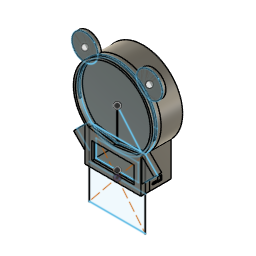
Data-visualization v7 (Autodesk Fusion 360 design; units mm, degrees)
Autodesk Fusion 360 part; units mm, degrees
sketch "Sketch1" plane through (0, 0, 0) normal (0, 1, 0) x (1, 0, 0)
  line L0 (49, -55) -> (-49, -55)
  line L1 (0, -15) -> (49, -15)
  line L2 (0, -15) -> (-49, -15)
  line L3 (-49, -55) -> (-49, -15)
  line L4 (49, -15) -> (49, -55)
  line L5 (65, -80) -> (-65, -80)
  line L6 (-65, -80) -> (-65, 80)
  line L7 (-65, 80) -> (65, 80)
  line L8 (65, 80) -> (65, -80)
  line L9 (65, -80) -> (-65, 80) construction
  line L10 (-65, -80) -> (65, 80) construction
  line L11 (0, -80) -> (0, -145)
  line L12 (0, -70) -> (65, -80)
  line L13 (0, -70) -> (-65, -80)
  circle A0 centre (0, -145) radius 91.9239
  line L14 (-65, 0) -> (65, 0)
  circle A1 centre (0, -145) radius 86.9239
  line L15 (65, -80) -> (93.2843, -51.7157)
  line L16 (93.2843, -51.7157) -> (65, -23.4315)
  line L17 (-65, -80) -> (-93.2843, -51.7157)
  line L18 (-93.2843, -51.7157) -> (-65, -23.4315)
  circle A2 centre (-75, -225) radius 30
  circle A3 centre (75, -225) radius 30
  circle A4 centre (0, -145) radius 2.5
  line L19 (0, -145) -> (0, -70)
  line L20 (0, -145) -> (56.14, -78.6369)
  point P0 (0, -15)
  dimension "d2" = 130
  dimension "d3" = 65
  dimension "d6" = -5
  dimension "d9" = 40
  dimension "d13" = 60
  dimension "d14" = 60
  dimension "d29" = 5
  constraint horizontal L0
  constraint coincident P0 L1.start
  constraint perpendicular L2 L3
  constraint perpendicular L0 L4
  constraint horizontal L5
  constraint perpendicular L5 L6
  constraint parallel L5 L7
  constraint parallel L6 L8
  constraint coincident L9 origin
  constraint coincident L10 origin
  constraint midpoint L5 L11.start
  constraint perpendicular L5 L11
  constraint coincident L11.end A0.centre
  constraint coincident L5.start A0
  constraint midpoint L6 L14.start
  constraint midpoint L8 L14.end
  constraint coincident L8 L16.end
  constraint perpendicular L15 L16
  constraint parallel L16 L17
  constraint coincident L6 L18.end
  constraint perpendicular L17 L18
  constraint concentric A0 A4
  constraint parallel L11 L19
  constraint coincident L12 L20.end
  constraint coincident A1 L20.end
  measures "d2" distance of L6.end L7.end
  measures "d3" distance of L11.start L11.end
  measures "d9" distance of L5.start L15.end
  measures "d13" diameter of A2
  measures "d14" diameter of A3
  measures "d29" diameter of A4
extrude "Extrude1" add sketch "Sketch1" along normal blind 10 contours L0 L1 L2 L3 L4 L6 L8 A0 L14 | L0 L12 L13 A0 A1 | L5 A0 A1 A3 | L5 L12 A1 | L5 L13 A1 | L5 A0 A1 A2 | L5 L11 A1 A2 A3 A4 L19 L20 | L5 A1 L20 | L5 L12 L19 L20 | L12 L13 A1 | L5 L13 A1 L19 | A0 A1 A2 | L5 L11 A4 L19 L20 | A0 A1 A3 | A1 A2 | A0 A1 A2 A3 | L11 A4 L19 L20 | L11 A4 L19 L20 | A1 A3 makes body 1
extrude "Extrude2" cut sketch "Sketch1" along normal blind 6 contours L5 L11 A1 A2 A3 A4 L19 L20 | L5 L11 A4 L19 L20 | A1 A2 | L11 A4 L19 L20 | L11 A4 L19 L20 | A1 A3 bodies 1
extrude "Extrude3" add sketch "Sketch1" along normal blind 10 contours L8 L15 L16 | L6 L17 L18 bodies 1
extrude "Extrude4" add sketch "Sketch1" along normal blind 6 contours A0 A3 bodies 1
extrude "Extrude5" add sketch "Sketch1" along normal blind 6 contours A0 A2 bodies 1
extrude "Extrude6" cut sketch "Sketch1" along normal blind 6 contours L5 A1 L20 | L5 L12 L19 L20 | L5 L13 A1 L19 bodies 1
extrude "Extrude7" add sketch "Sketch1" against normal blind 10 contours L0 L1 L2 L3 L4 L6 L8 A0 L14 | L0 L12 L13 A0 A1 | L5 A0 A1 A3 | L5 L12 A1 | L5 L13 A1 | L5 A0 A1 A2 | A0 A1 A2 | A0 A1 A3 | A0 A1 A2 A3 bodies 1
extrude "Extrude8" add sketch "Sketch1" against normal blind 10 contours L12 L13 A1 bodies 1
sketch "Sketch2" plane through (0, 0, 360) normal (0, 0, -1) x (1, 0, 0)
  line L0 (-200, 0) -> (200, 0)
  line L1 (200, 0) -> (200, 4.5)
  line L2 (200, 4.5) -> (-200, 4.5)
  line L3 (-200, 4.5) -> (-200, 0)
  line L4 (-200, 4.5) -> (200, 4.5)
  line L5 (200, 4.5) -> (200, 0)
  line L6 (200, 0) -> (-200, 0)
  line L7 (-200, 0) -> (-200, 4.5)
  constraint horizontal L4
  constraint vertical L5
  constraint horizontal L6
  constraint vertical L7
  constraint coincident L0.end L1.start
  constraint coincident L2.end L3.start
extrude "Extrude10" cut sketch "Sketch2" along normal blind 240 bodies 1
extrude "Extrude11" cut sketch "Sketch1" along normal blind 10 contours L11 A4 L19 L20 | L11 A4 L19 L20 bodies 1
extrude "Extrude12" add sketch "Sketch1" against normal blind 8 contours L8 L15 L16 bodies 1
extrude "Extrude13" add sketch "Sketch1" against normal blind 8 contours L6 L17 L18 bodies 1
sketch "Sketch4" plane through (0, 10, 0) normal (0, 1, 0) x (-1, 0, 0)
  circle A0 centre (0, 145) radius 2.5
  line L0 (49, 15) -> (-49, 15)
  line L1 (-49, 15) -> (-49, 55)
  line L2 (-49, 55) -> (49, 55)
  line L3 (49, 55) -> (49, 15)
  arc A1 (65, 80) -> (-65, 80) centre (0, 145) ccw
  line L4 (-65, 80) -> (-93.2843, 51.7157)
  line L5 (-93.2843, 51.7157) -> (-65, 23.4315)
  line L6 (-65, 23.4315) -> (-65, 0)
  line L7 (-65, 0) -> (65, 0)
  line L8 (65, 0) -> (65, 23.4315)
  line L9 (65, 23.4315) -> (93.2843, 51.7157)
  line L10 (93.2843, 51.7157) -> (65, 80)
  line L11 (-65, 80) -> (65, 80)
  line L12 (65, 80) -> (65, 0)
  line L13 (65, 0) -> (-65, 0)
  line L14 (-65, 0) -> (-65, 80)
  circle A2 centre (0, 145) radius 91.9239
  constraint horizontal L11
  constraint vertical L12
  constraint horizontal L13
  constraint vertical L14
  constraint coincident L7.end L8.start
  constraint coincident A1.end L4.start
  constraint concentric A0 A2
extrude "Extrude14" add sketch "Sketch4" along normal blind 50 separate body contours L0 L1 L2 L3 L6 L7 L8 L12 L13 L14 A2 | L0 L1 L2 L3 A2 | L2 A2 | L2 L11 A2 | A1 L11 A2 makes body 2
move_face "OffsetFaces1" offset 50 1 faces at (-2.4504, 43.3333, 144.5046) on bodies 2
sketch "Sketch5" plane through (0, 10, 0) normal (0, -1, 0) x (1, 0, 0)
  line L0 (-65, 80) -> (-65, 0)
  line L1 (-65, 0) -> (65, 0)
  line L2 (65, 0) -> (65, 80)
  arc A0 (65, 80) -> (-65, 80) centre (0, 145) ccw
  circle A1 centre (0, 145) radius 85
  line L3 (-60, 84.792) -> (-60, 5)
  line L4 (-60, 84.792) -> (60, 84.792)
  line L5 (60, 84.792) -> (60, 5)
  line L6 (60, 5) -> (-60, 5)
  line L7 (-60, 5) -> (-60, 84.792)
  dimension "d39" = 170
  dimension "d40" = -5
  constraint concentric A0 A1
  constraint coincident A1 L3.start
  constraint horizontal L4
  constraint vertical L5
  constraint horizontal L6
  constraint vertical L7
  measures "d39" diameter of A1
extrude "Extrude15" cut sketch "Sketch5" against normal blind 45 contours A1 L4 picked at (-9.4952, 166.9681) bodies 2
extrude "Extrude16" cut sketch "Sketch5" against normal blind 45 contours A1 L4 | A1 L3 L5 L6 L7 picked at (16.9474, 82.1553) bodies 2
sketch "Sketch6" plane through (0, 10, 0) normal (0, 1, 0) x (-1, 0, 0)
  circle A0 centre (0, 145) radius 2.5
  line L0 (49, 15) -> (-49, 15)
  line L1 (-49, 15) -> (-49, 55)
  line L2 (-49, 55) -> (49, 55)
  line L3 (49, 55) -> (49, 15)
  arc A1 (65, 80) -> (-65, 80) centre (0, 145) ccw
  line L4 (-65, 80) -> (-93.2843, 51.7157)
  line L5 (-93.2843, 51.7157) -> (-65, 23.4315)
  line L6 (-65, 23.4315) -> (-65, 0)
  line L7 (-65, 0) -> (65, 0)
  line L8 (65, 0) -> (65, 23.4315)
  line L9 (65, 23.4315) -> (93.2843, 51.7157)
  line L10 (93.2843, 51.7157) -> (65, 80)
  line L11 (65, 0) -> (-65, 0)
  line L12 (-65, 0) -> (-65, 80)
  line L13 (-65, 80) -> (65, 80)
  line L14 (65, 80) -> (65, 0)
  line L15 (61, 4) -> (-61, 4)
  line L16 (-61, 4) -> (-61, 76)
  line L17 (-61, 76) -> (61, 76)
  line L18 (61, 76) -> (61, 4)
  line L19 (0, 66) -> (61, 66)
  line L20 (0, 66) -> (-61, 66)
  line L21 (-65, 70) -> (65, 70)
  line L22 (-65, 70) -> (-62, 70)
  line L23 (-62, 70) -> (-62, 34)
  line L24 (-62, 34) -> (-65, 34)
  line L25 (-65, 34) -> (-65, 70)
  line L26 (65, 70) -> (62, 70)
  line L27 (62, 70) -> (62, 34)
  line L28 (62, 34) -> (65, 34)
  line L29 (65, 34) -> (65, 70)
  dimension "d45" = 4
  dimension "d52" = 3
  dimension "d53" = 36
  dimension "d54" = 3
  dimension "d55" = 36
  constraint horizontal L11
  constraint vertical L12
  constraint horizontal L13
  constraint vertical L14
  constraint coincident A1.end L4.start
  constraint coincident L7.end L8.start
  constraint coincident L18 L19.end
  constraint perpendicular L18 L19
  constraint coincident L16 L20.end
  constraint perpendicular L16 L20
  constraint coincident L12 L21.start
  constraint coincident L14 L21.end
  constraint perpendicular L14 L21
  constraint horizontal L22
  constraint vertical L23
  constraint horizontal L24
  constraint vertical L25
  constraint horizontal L26
  constraint vertical L27
  constraint horizontal L28
  constraint vertical L29
  measures "d52" distance of L21.start L22.end
  measures "d53" distance of L21.start L24.end
  measures "d8" distance of L21.end L26.end
  measures "d8" distance of L21.end L28.end
extrude "Extrude17" cut sketch "Sketch6" against normal blind 15 contours L15 L16 L18 L19 L20 bodies 1
extrude "Extrude18" cut sketch "Sketch6" against normal blind 10 contours L14 L21 L26 L27 L28 L29 | L12 L21 L22 L23 L24 L25 bodies 1
extrude "Extrude19" add sketch "Sketch6" against normal blind 9.9 contours L14 L21 L26 L27 L28 L29 | L12 L21 L22 L23 L24 L25 bodies 2
move_face "OffsetFaces2" offset -0.2 1 faces at (-65, 6.6667, 58) on bodies 1
sketch "Sketch7" plane through (65, 0, 0) normal (1, 0, 0) x (0, 1, 0)
  line L0 (10, 34) -> (10, 0)
  line L1 (10, 0) -> (60, 0)
  line L2 (60, 0) -> (60, 80)
  line L3 (60, 80) -> (10, 80)
  line L4 (10, 80) -> (10, 70)
  line L5 (10, 70) -> (0.1, 70)
  line L6 (0.1, 70) -> (0.1, 34)
  line L7 (0.1, 34) -> (10, 34)
  line L8 (38.3, 19.65) -> (29.1, 19.65)
  line L9 (29.1, 19.65) -> (29.1, 8.45)
  line L10 (29.1, 8.45) -> (38.3, 8.45)
  line L11 (38.3, 8.45) -> (38.3, 19.65)
  line L12 (38.3, 19.65) -> (29.1, 8.45) construction
  line L13 (29.1, 19.65) -> (38.3, 8.45) construction
  line L14 (27.8, 14.05) -> (16.2, 14.05)
  line L15 (16.2, 14.05) -> (16.2, 9.25)
  line L16 (16.2, 9.25) -> (27.8, 9.25)
  line L17 (27.8, 9.25) -> (27.8, 14.05)
  line L18 (27.8, 14.05) -> (16.2, 9.25) construction
  line L19 (16.2, 14.05) -> (27.8, 9.25) construction
  point P0 (33.7, 14.05)
  point P1 (22, 11.65)
  dimension "d71" = 9.2
  dimension "d72" = 11.2
  dimension "d73" = 11.6
  dimension "d74" = 4.8
  constraint horizontal L8
  constraint perpendicular L8 L9
  constraint parallel L8 L10
  constraint parallel L9 L11
  constraint coincident L12 P0
  constraint coincident L13 P0
  constraint horizontal L14
  constraint perpendicular L14 L15
  constraint parallel L14 L16
  constraint parallel L15 L17
  constraint coincident L18 P1
  constraint coincident L19 P1
  measures "d71" distance of L9.end L10.end
  measures "d72" distance of L8.end L9.end
  measures "d73" distance of L15.end L16.end
  measures "d74" distance of L14.end L15.end
extrude "Extrude20" cut sketch "Sketch7" against normal blind 5 contours L8 L9 L10 L11 | L14 L15 L16 L17 bodies 2
fillet "Fillet1" radius 0.5 4 edges at (62.5, 38.3, 19.65) (62.5, 38.3, 8.45) (62.5, 29.1, 8.45) (62.5, 29.1, 19.65) on bodies 2
fillet "Fillet2" radius 1.8 4 edges at (62.5, 27.8, 14.05) (62.5, 27.8, 9.25) (62.5, 16.2, 14.05) (62.5, 16.2, 9.25) on bodies 2
sketch "Sketch8" plane through (60, 0, 0) normal (-1, 0, 0) x (0, -1, 0)
  line L0 (-37.8, 19.65) -> (-29.6, 19.65)
  arc A0 (-29.1, 19.15) -> (-29.6, 19.65) centre (-29.6, 19.15) ccw
  line L1 (-29.1, 19.15) -> (-29.1, 8.95)
  arc A1 (-29.6, 8.45) -> (-29.1, 8.95) centre (-29.6, 8.95) ccw
  line L2 (-29.6, 8.45) -> (-37.8, 8.45)
  arc A2 (-38.3, 8.95) -> (-37.8, 8.45) centre (-37.8, 8.95) ccw
  line L3 (-38.3, 8.95) -> (-38.3, 19.15)
  arc A3 (-37.8, 19.65) -> (-38.3, 19.15) centre (-37.8, 19.15) ccw
  line L4 (-26, 14.05) -> (-18, 14.05)
  arc A4 (-16.2, 12.25) -> (-18, 14.05) centre (-18, 12.25) ccw
  line L5 (-16.2, 12.25) -> (-16.2, 11.05)
  arc A5 (-18, 9.25) -> (-16.2, 11.05) centre (-18, 11.05) ccw
  line L6 (-18, 9.25) -> (-26, 9.25)
  arc A6 (-27.8, 11.05) -> (-26, 9.25) centre (-26, 11.05) ccw
  line L7 (-27.8, 11.05) -> (-27.8, 12.25)
  arc A7 (-26, 14.05) -> (-27.8, 12.25) centre (-26, 12.25) ccw
  line L8 (-10, 5) -> (-10, 84.792)
  line L9 (-10, 84.792) -> (-55, 84.792)
  line L10 (-55, 84.792) -> (-55, 5)
  line L11 (-55, 5) -> (-10, 5)
  line L12 (-10, 5) -> (-46, 5)
  line L13 (-46, 5) -> (-46, 23)
  line L14 (-46, 23) -> (-10, 23)
  line L15 (-10, 23) -> (-10, 5)
  dimension "d81" = 18
  constraint horizontal L12
  constraint vertical L13
  constraint horizontal L14
  constraint vertical L15
  constraint coincident L8.start L11.end
  measures "d81" distance of L8.start L14.end
extrude "Extrude21" cut sketch "Sketch8" against normal blind 2 contours L8 L11 L12 L13 L14 L15 bodies 2
copy_body "CopyPasteBodies1" bodies 1 makes body 3
move_face "OffsetFaces3" offset -10 2 faces at (-60.4621, 6, 228.0645) (78.9951, 6, 210.6898) on bodies 3
extrude "Extrude22" add sketch "Sketch1" along normal blind 8 separate body contours A0 A2 | A0 A3 makes body 4 at (-60.4621, 0, 228.0645) makes body 5 at (78.9951, 0, 210.6898)
sketch "Sketch9" plane through (0, 0, 120) normal (0, 0, 1) x (-1, 0, 0)
  line L0 (-88.459, 4.5) -> (-88.459, 0)
  line L1 (-88.459, 0) -> (-83.2512, 0)
  line L2 (-83.2512, 0) -> (-83.2512, 4.5)
  line L3 (-83.2512, 4.5) -> (-88.459, 4.5)
  line L4 (56.14, 0) -> (-56.14, 0)
  line L5 (-56.14, 0) -> (-56.14, 4.5)
  line L6 (-56.14, 4.5) -> (56.14, 4.5)
  line L7 (56.14, 4.5) -> (56.14, 0)
  constraint horizontal L4
  constraint vertical L5
  constraint horizontal L6
  constraint vertical L7
extrude "Extrude23" cut sketch "Sketch9" against normal blind 50 contours L4 L5 L6 L7 bodies 3
hidden bodies 1
named bodies: "frontcover(use)", "mainbody(use)", "frontcover(use) (1)", "ear_a", "ear_b"
